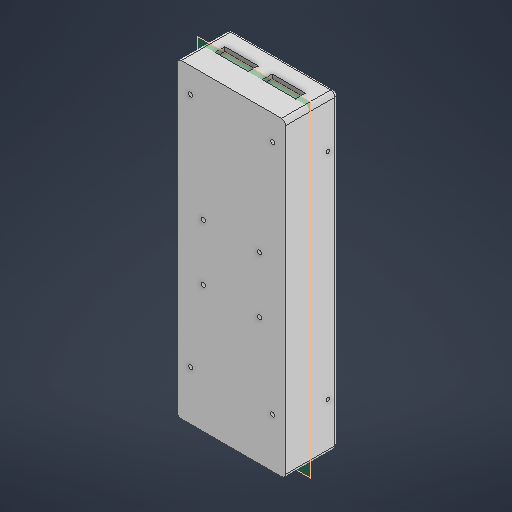
# Autodesk Inventor part: Part17
Saved by Autodesk Inventor 2025.3 (Build 293356030, 356C)
## iProperties
Created: 2025-09-03
Part Number: Part17
Material: Generic
Document SubType Name: Modeling
Designer: river
Density: 1 g/cm^3
Appearance: Default
Author: river
Autodesk Inventor part; units mm, degrees
ref_plane "YZ Plane" through (0, 0, 0) normal (1, 0, 0) x (0, 1, 0)
ref_plane "XZ Plane" through (0, 0, 0) normal (0, 1, 0) x (-1, 0, 0)
ref_plane "XY Plane" through (0, 0, 0) normal (0, 0, 1) x (1, 0, 0)
ref_plane "Work Plane1" through (0, 0, 0) normal (0, 0, 1) x (1, 0, 0)
sketch "Sketch1" plane through (0, 0, 0) normal (0, 0, 1) x (1, 0, 0)
  line L0 (33.655, -97.47) -> (-33.655, -97.47) construction
  line L1 (33.655, 97.47) -> (33.655, -97.47) construction
  line L2 (-33.655, 97.47) -> (33.655, 97.47) construction
  line L3 (-33.655, -97.47) -> (-33.655, 97.47) construction
  circle A0 centre (-29.0882, 92.7751) radius 1.5 projected
  circle A1 centre (29.3416, 92.7751) radius 1.5 projected
  circle A2 centre (-29.0882, -75.1694) radius 1.5 projected
  circle A3 centre (29.3416, -75.297) radius 1.5 projected
sketch "Sketch2" plane through (0, 0, 0) normal (0, 0, 1) x (1, 0, 0)
  circle A0 centre (29.3416, -75.297) radius 1.5 projected
  line L0 (33.655, 97.47) -> (33.655, -97.47) construction
  line L1 (33.655, -97.47) -> (-33.655, -97.47) construction
  circle A1 centre (-29.0882, -75.1694) radius 1.5 projected
  line L2 (-33.655, -97.47) -> (-33.655, 97.47) construction
  line L3 (-33.655, 97.47) -> (33.655, 97.47) construction
  circle A2 centre (-29.0882, 92.7751) radius 1.5 projected
  circle A3 centre (29.3416, 92.7751) radius 1.5 projected
  circle A4 centre (29.3416, -75.297) radius 4.5
  circle A5 centre (29.3416, 92.7751) radius 4.5
  circle A6 centre (-29.0882, -75.1694) radius 4.5
  circle A7 centre (-29.0882, 92.7751) radius 4.5
  line L4 (-35.655, 107.47) -> (35.655, 107.47)
  line L5 (35.655, 107.47) -> (35.655, -107.47)
  line L6 (35.655, -107.47) -> (-35.655, -107.47)
  line L7 (-35.655, -107.47) -> (-35.655, 107.47)
  line L8 (-35.655, 107.47) -> (35.655, -107.47) construction
  line L9 (35.655, 107.47) -> (-35.655, -107.47) construction
  line L10 (-38.655, -110.47) -> (38.655, -110.47)
  line L11 (38.655, -110.47) -> (38.655, 110.47)
  line L12 (38.655, 110.47) -> (-38.655, 110.47)
  line L13 (-38.655, 110.47) -> (-38.655, -110.47)
  line L14 (-33.655, 0) -> (33.655, 0) construction
  line L15 (0, 97.47) -> (0, -97.47) construction
  circle A8 centre (-20, 20) radius 1.5
  circle A9 centre (-20, -20) radius 1.5
  circle A10 centre (20, 20) radius 1.5
  circle A11 centre (20, -20) radius 1.5
  point P0 (0, 0)
  dimension "d3" = 9
  dimension "d13" = 2
  dimension "d14" = 10
  dimension "d15" = 3
  dimension "d86" = 3
  dimension "d87" = 40
  dimension "d88" = 40
  constraints: 24 end point, 8 centre point, 6 midpoint, 4 coincident, 4 parallel, 3 equal radius, 3 symmetric about line, 2 perpendicular, 1 horizontal, 6 other
  measures "d3" diameter of A4
  measures "d13" distance between parallel lines of L5 L0
  measures "d14" distance between parallel lines of L6 L1
  measures "d15" distance between parallel lines of L6 L10
  measures "d86" diameter of A8
  measures "d87" distance of A9.centre A8.centre
  measures "d88" distance of A10.centre A8.centre
extrude "Extrusion1" add sketch "Sketch2" along normal blind 3 contours A4 | A5 | A6 | A7
extrude "Extrusion2" add sketch "Sketch2" along normal blind 3 from surface at 3 contours A4 | A5 | A6 | A7 | L4 L5 L6 L7 | L13 L12 L11 L10
extrude "Extrusion3" add sketch "Sketch2" against normal blind 32 from surface at 3 contours L13 L12 L11 L10
fillet "Fillet1" radius 3 4 edges at (-38.655, -110.47, -11.5) (38.655, -110.47, -11.5) (38.655, 110.47, -11.5) (-38.655, 110.47, -11.5)
ref_plane "Work Plane2" through (35.655, -107.47, -11) normal (0, 0, -1) x (-1, 0, 0)
sketch "Sketch4" plane through (35.655, -107.47, -11) normal (0, 0, -1) x (-1, 0, 0)
  line L0 (0, 214.94) -> (0, 0) construction
  line L1 (71.31, 214.94) -> (0, 214.94) construction
  line L2 (71.31, 0) -> (71.31, 214.94) construction
  line L3 (0, 206.94) -> (71.31, 206.94)
  line L4 (71.31, 206.94) -> (71.31, 214.94)
  line L5 (71.31, 214.94) -> (0, 214.94)
  line L6 (0, 214.94) -> (0, 206.94)
  line L7 (35.655, 206.94) -> (35.655, 214.94) construction
  line L8 (7, 206.94) -> (7, 214.94)
  line L9 (30.655, 214.94) -> (30.655, 206.94)
  circle A0 centre (35.655, 210.94) radius 1.25
  circle A1 centre (3.5, 210.94) radius 1.25
  line L10 (64.31, 206.94) -> (64.31, 214.94)
  line L11 (40.655, 214.94) -> (40.655, 206.94)
  circle A2 centre (67.81, 210.94) radius 1.25
  line L12 (7, 214.94) -> (7, 228.5816)
  line L13 (7, 228.5816) -> (30.655, 228.5816)
  line L14 (30.655, 228.5816) -> (30.655, 214.94)
  line L15 (40.655, 214.94) -> (40.655, 228.5816)
  line L16 (40.655, 228.5816) -> (64.31, 228.5816)
  line L17 (64.31, 228.5816) -> (64.31, 214.94)
  point P0 (35.655, 107.47)
  dimension "d27" = 8
  dimension "d28" = 7
  dimension "d29" = 5
  dimension "d30" = 2.5
  dimension "d31" = 4
  dimension "d32" = 3.5
  constraints: 30 end point, 7 point on line, 5 perpendicular, 5 symmetric about line, 3 centre point, 3 midpoint, 3 parallel, 2 vertical, 1 equal radius, 1 horizontal, 1 other
  measures "d27" distance between parallel lines of L1 L3
  measures "d28" distance between parallel lines of L0 L8
  measures "d29" distance between parallel lines of L9 L7
  measures "d30" diameter of A0
  measures "d31" distance from line of L1 A1.centre
  measures "d32" distance from line of L6 A1.centre
extrude "Extrusion5" cut sketch "Sketch4" along normal blind 7 contours L12 L13 L14 L5 | L15 L16 L17 L5
extrude "Extrusion6" add sketch "Sketch4" against normal up to surface (14 mm away) contours L6 L5 L8 L3 | L8 L5 L9 L3 | L9 L5 L11 L3 | L11 L5 L10 L3 | L10 L5 L4 L3 | A0 | A1 | A2
extrude "Extrusion7" cut sketch "Sketch4" against normal blind 5 contours A0 | A1 | A2
sketch "Sketch5" plane through (-38.655, -107.47, -29) normal (-1, 0, 0) x (0, 0, 1)
  line L0 (18, 214.94) -> (18, 206.94) projected
  line L1 (18, 206.94) -> (32, 206.94) projected
  line L2 (18, 206.94) -> (19, 207.94)
  line L3 (19, 207.94) -> (18, 208.94)
  line L4 (18, 208.94) -> (19, 209.94)
  line L5 (19, 209.94) -> (18, 210.94)
  line L6 (18, 210.94) -> (19, 211.94)
  line L7 (19, 211.94) -> (18, 212.94)
  line L8 (18, 212.94) -> (19, 213.94)
  line L9 (19, 213.94) -> (18, 214.94)
  point P0 (29, 107.47)
  point P1 (18, 210.94)
  point P2 (18, 208.94)
  dimension "d39" = 1
  dimension "d40" = 1
  dimension "d41" = 1
  dimension "d44" = 2
  constraints: 16 end point, 1 point on line, 1 vertical, 15 other
  measures "d39" horizontal distance of L2.end L0.end
  measures "d40" horizontal distance of L0.end L2.end
  measures "d41" horizontal distance of L3.end L2.end
  measures "d44" distance of L0.end L4.start
extrude "Extrusion8" cut sketch "Sketch5" against normal up to surface (71.31 mm away) from surface at -3
extrude "Extrusion9" add sketch "Sketch4" against normal blind 10 contours L6 L5 L8 L3 | L9 L5 L11 L3 | L10 L5 L4 L3
mirror "Mirror1" about plane through (0, 0, 0) normal (0, 1, 0) of "Extrusion8", "Extrusion6", "Extrusion5", "Extrusion9", "Extrusion7"
extrude "Extrusion10" add sketch "Sketch4" along normal blind 3 separate body contours L6 L5 L8 L3 | L8 L5 L9 L3 | L9 L5 L11 L3 | L11 L5 L10 L3 | L10 L5 L4 L3
sketch "Sketch6" plane through (35.655, -107.47, -14) normal (0, 0, -1) x (-1, 0, 0)
  line L0 (0, 206.94) -> (71.31, 206.94) projected
  line L1 (71.31, 206.94) -> (71.31, 214.94) projected
  line L2 (71.31, 214.94) -> (0, 214.94) projected
  line L3 (0, 214.94) -> (0, 206.94) projected
  circle A0 centre (35.655, 210.94) radius 1.25 projected
  circle A1 centre (67.81, 210.94) radius 1.25 projected
  circle A2 centre (3.5, 210.94) radius 1.25 projected
  circle A3 centre (3.5, 210.94) radius 3
  line L4 (0, 213.94) -> (71.31, 213.94)
  circle A4 centre (35.655, 210.94) radius 3
  circle A5 centre (67.81, 210.94) radius 3
  line L5 (31.655, 213.94) -> (31.655, 206.94)
  line L6 (39.655, 213.94) -> (39.655, 206.94)
  line L7 (7.5, 206.94) -> (7.5, 213.94)
  line L8 (71.31, 206.94) -> (0, 206.94) projected
  line L9 (63.81, 206.94) -> (63.81, 213.94)
  point P0 (35.655, 107.47)
  dimension "d55" = 6
  dimension "d56" = 4
  dimension "d57" = 4
  dimension "d58" = 4
  dimension "d59" = 4
  constraints: 10 end point, 10 point on line, 3 centre point, 3 coincident, 3 perpendicular, 2 equal radius, 2 vertical, 1 tangent
  measures "d55" diameter of A3
  measures "d56" distance from line of L5 A0.centre
  measures "d57" distance from line of A0.centre L6
  measures "d58" distance from line of L7 A2.centre
  measures "d59" distance from line of L9 A1.centre
extrude "Extrusion11" add sketch "Sketch6" along normal blind 6 contours L7 L4 L5 L0 | L3 L2 L1 L4 | L6 L4 L9 L0 bodies 2
chamfer "Chamfer1" distance 6 angle 45 2 edges at (16.0775, 99.47, -20) (-16.0775, 99.47, -20)
thicken "Thicken1" operation cut thickness 0.4 both sides no extend neighbours no toward (1, 0, 0) bodies 2 faces at (-35.655, 104.47, -12) (-11.885, 107.47, -14) (35.655, 104.47, -12)
fillet "Fillet2" radius 2 4 edges at (35.255, 106.77, -20) (35.255, 99.47, -12.5) (-35.255, 106.77, -20) (-35.255, 99.47, -12.5)
fillet "Fillet3" radius 2 4 edges at (-4, 106.47, -17) (28.155, 106.47, -17) (4, 106.47, -17) (-28.155, 106.47, -17)
sketch "Sketch7" plane through (35.655, 110.47, -29) normal (0, 0, -1) x (-1, 0, 0)
  arc A0 (74.31, -3) -> (71.31, 0) centre (71.31, -3) ccw projected
  line L0 (71.31, 0) -> (0, 0) projected
  arc A1 (0, 0) -> (-3, -3) centre (0, -3) ccw projected
  line L1 (-3, -3) -> (-3, -217.94) projected
  arc A2 (-3, -217.94) -> (0, -220.94) centre (0, -217.94) ccw projected
  line L2 (0, -220.94) -> (71.31, -220.94) projected
  arc A3 (71.31, -220.94) -> (74.31, -217.94) centre (71.31, -217.94) ccw projected
  line L3 (74.31, -217.94) -> (74.31, -3) projected
  line L4 (0, -217.94) -> (0, -3) projected
  line L5 (0, -3) -> (71.31, -3) projected
  line L6 (71.31, -3) -> (71.31, -217.94) projected
  line L7 (71.31, -217.94) -> (0, -217.94) projected
  line L8 (0.5, -3.5) -> (0.5, -217.44)
  line L9 (0.5, -217.44) -> (70.81, -217.44)
  line L10 (70.81, -217.44) -> (70.81, -3.5)
  line L11 (70.81, -3.5) -> (0.5, -3.5)
  point P0 (35.655, -110.47)
  dimension "d69" = 0.5
  constraints: 8 end point, 3 other
  measures "d69" distance between parallel lines of L4 L8
extrude "Extrusion12" add sketch "Sketch7" against normal blind 1 separate body contours L11 L10 L9 L8
extrude "Extrusion13" add sketch "Sketch7" along normal blind 2 contours L3 A3 L2 A2 L1 A1 L0 A0 | L4 L5 L6 L7 | L11 L10 L9 L8 bodies 3
fillet "Fillet4" radius 2 8 edges at (-37.7763, 109.5913, -31) (0, 110.47, -31) (37.7763, 109.5913, -31) (38.655, 0, -31) (37.7763, -109.5913, -31) (0, -110.47, -31) (-37.7763, -109.5913, -31) (-38.655, 0, -31)
sketch "Sketch8" plane through (0, 0, 0) normal (1, 0, 0) x (0, 1, 0)
  line L0 (106.97, -28) -> (-106.97, -28) projected
  line L1 (-83.9709, -28) -> (-83.9709, -20)
  line L2 (-83.9709, -20) -> (-68.9709, -20)
  line L3 (-68.9709, -20) -> (-68.9709, -28)
  circle A0 centre (-76.4709, -24) radius 1.25
  line L4 (-83.9709, -24) -> (-68.9709, -24) construction
  line L5 (-76.4709, -20) -> (-76.4709, -28) construction
  point P0 (0, 0)
  dimension "d75" = 15
  dimension "d76" = 8
  dimension "d77" = 2.5
  constraints: 10 end point, 4 midpoint, 3 perpendicular, 3 point on line, 1 centre point, 1 vertical
  measures "d75" distance of L1.end L2.end
  measures "d76" distance of L1.start L1.end
  measures "d77" diameter of A0
extrude "Extrusion14" add sketch "Sketch8" along normal blind 4 from surface at -35.155 bodies 3
fillet "Fillet5" radius 3 4 edges at (-33.155, -83.9709, -20) (-33.155, -83.9709, -28) (-33.155, -68.9709, -20) (-33.155, -68.9709, -28)
chamfer "Chamfer2" distance 3 angle 45 3 edges at (-31.155, -67.4709, -28) (-31.155, -85.4709, -28) (-31.155, -76.4709, -28)
mirror "Mirror2" about plane through (0, 0, 0) normal (1, 0, 0) of "Extrusion14", "Chamfer2", "Fillet5" bodies 3
mirror "Mirror3" about plane through (0, 0, 0) normal (0, 1, 0) of "Extrusion14", "Chamfer2", "Fillet5", "Mirror2" bodies 3
extrude "Extrusion15" cut sketch "Sketch8" against normal blind 4 from surface at -35.655 contours A0 bodies 1
mirror "Mirror4" about plane through (0, 0, 0) normal (1, 0, 0) of "Extrusion15" bodies 1
mirror "Mirror5" about plane through (0, 0, 0) normal (0, 1, 0) of "Extrusion15", "Mirror4" bodies 1
equation "\"d31\" = 0.5 * d27"
equation "\"d32\" = 0.5 * d28"
equation "\"d57\" = d56"
body "Solid1"
body "Solid2"
body "Solid3"
